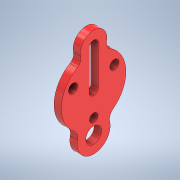
# Autodesk Inventor part: hw11
Saved by Autodesk Inventor 2021 (Build 250183000, 183)
## iProperties
Created: 2022-04-30
Part Number: hw11
Material: Generic
Document SubType Name: Modeling
Designer: authe
Density: 1 g/cm^3
Appearance: Light Red
Author: authe
Autodesk Inventor part; units mm, degrees
ref_plane "YZ Plane" through (0, 0, 0) normal (1, 0, 0) x (0, 1, 0)
ref_plane "XZ Plane" through (0, 0, 0) normal (0, 1, 0) x (-1, 0, 0)
ref_plane "XY Plane" through (0, 0, 0) normal (0, 0, 1) x (1, 0, 0)
sketch "Sketch1" plane through (0, 0, 0) normal (1, 0, 0) x (0, 1, 0)
  arc A0 (97.7884, -35.051) -> (97.7884, 35.051) centre (106, 0) ccw
  arc A1 (75.9623, 44.4267) -> (97.7884, 35.051) centre (93.2264, 54.5237) ccw
  arc A2 (97.7884, -35.051) -> (75.9623, -44.4267) centre (93.2264, -54.5237) ccw
  arc A3 (-95.7901, 43.8265) -> (-95.7901, -43.8265) centre (-106, 0) ccw
  arc A4 (-95.7901, 43.8265) -> (-70.1803, 53.0916) centre (-90.1179, 68.1745) ccw
  arc A5 (-70.1803, -53.0916) -> (-95.7901, -43.8265) centre (-90.1179, -68.1745) ccw
  arc A6 (75.9623, 44.4267) -> (-70.1803, 53.0916) centre (0, 0) ccw
  arc A7 (-70.1803, -53.0916) -> (75.9623, -44.4267) centre (0, 0) ccw
  circle A8 centre (0, 0) radius 65
  circle A9 centre (-65, 0) radius 11.5
  circle A10 centre (-106, 0) radius 21.5
  arc A11 (0, 12.5) -> (0, -12.5) centre (0, 0) ccw
  arc A12 (106, -12.5) -> (106, 12.5) centre (106, 0) ccw
  line L0 (106, 12.5) -> (0, 12.5)
  line L1 (0, -12.5) -> (106, -12.5)
  line L2 (-12.5, 0) -> (-53.5, 0)
  circle A13 centre (32.5, 56.2917) radius 12.5
  circle A14 centre (32.5, -56.2917) radius 12.5
  dimension "d27" = 23
  dimension "d19" = 12.5
  dimension "d20" = 36
  dimension "d21" = 106
  dimension "d22" = 212
  dimension "d23" = 25
  dimension "d24" = 25
  dimension "d25" = 43
  dimension "d26" = 45
  dimension "d28" = 88
  dimension "d29" = 25
  dimension "d30" = 25
  dimension "d31" = 20
  dimension "d32" = 20
  constraints: 21 point on circle, 13 centre point, 6 end point, 5 tangent, 4 coincident, 2 horizontal alignment, 1 horizontal, 1 parallel, 4 other
  measures "d19" radius of A12
  measures "d20" radius of A0
  measures "d21" distance of L0.start L0.end
  measures "d22" distance of A3.centre A0.centre
  measures "d23" diameter of A14
  measures "d24" diameter of A13
  measures "d25" diameter of A10
  measures "d26" radius of A3
  measures "d28" radius of A6
  measures "d29" radius of A4
  measures "d30" radius of A5
  measures "d31" radius of A2
  measures "d32" radius of A1
extrude "Extrusion1" add sketch "Sketch1" along normal blind 20 contours A2 A7 A5 A3 A4 A6 A1 A0 | L0 A11 L2 A9 A8 A13 | A8 A14 A9 L2 A11 L1
body "Solid1"
